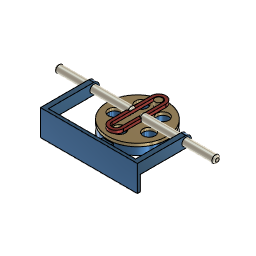
Scotch Yoke (Autodesk Fusion 360 design; units mm, degrees)
Autodesk Fusion 360 part; units mm, degrees
sketch "Sketch1" plane through (0, 0, 0) normal (0, 0, 1) x (1, 0, 0)
  circle A0 centre (0, 0) radius 49
  circle A1 centre (0, 35) radius 6
  line L0 (7, -35) -> (7, 35)
  arc A2 (7, 35) -> (-7, 35) centre (0, 35) ccw
  line L1 (-7, 35) -> (-7, -35)
  arc A3 (-7, -35) -> (7, -35) centre (0, -35) ccw
  line L2 (0, -35) -> (0, 35) construction
  line L3 (12, -35) -> (12, 35)
  arc A4 (12, 35) -> (-12, 35) centre (0, 35) ccw
  line L4 (-12, 35) -> (-12, -35)
  arc A5 (-12, -35) -> (12, -35) centre (0, -35) ccw
  dimension "d1" = 98
  dimension "d2" = 12
  dimension "d3" = 35
  dimension "d4" = 14
  dimension "d5" = 5
  constraint coincident A0.centre origin
  constraint vertical A0.centre A1.centre
  constraint tangent L0 A2
  constraint tangent A2 L1
  constraint parallel L0 L1
  constraint tangent L1 A3
  constraint tangent L0 A3
  constraint coincident A1.centre A2.centre
  constraint vertical L2
  constraint midpoint L2 A0.centre
  measures "d1" diameter of A0
  measures "d2" diameter of A1
  measures "d3" distance of A0.centre A1.centre
  measures "d4" diameter of A2
extrude "Extrude1" add sketch "Sketch1" against normal blind 5 contours A0 | A1 | L0 A2 L1 A3 | L3 A4 L4 A5 makes body 1
extrude "Extrude2" add sketch "Sketch1" along normal blind 10 contours A1 bodies 1
extrude "Extrude3" add sketch "Sketch1" along normal blind 5 separate body contours L3 A4 L4 A5 makes body 2
move_body "Align1" bodies 2 to x (1, 0, 0) y (0, 1, 0) z (0, 0, 1) at (0, 0, 5)
sketch "Sketch2" plane through (12, 0, 0) normal (1, 0, 0) x (0, 1, 0)
  line L0 (-35, 5) -> (35, 5)
  line L1 (35, 5) -> (35, 10)
  line L2 (35, 10) -> (-35, 10)
  line L3 (-35, 10) -> (-35, 5)
  line L4 (0, 5) -> (0, 7.5)
  circle A0 centre (0, 7.5) radius 6
  dimension "d12" = 2.5
  dimension "d13" = 12
  constraint midpoint L0 L4.start
  constraint perpendicular L2 L4
  constraint coincident L4.end A0.centre
  measures "d12" distance of L4.start L4.end
  measures "d13" diameter of A0
extrude "Extrude4" add sketch "Sketch2" along normal blind 60 separate body contours L0 L2 A0 | L0 A0 | L2 A0 makes body 3
extrude "Extrude5" add sketch "Sketch2" against normal blind 5 contours L0 A0 | L2 A0 bodies 3
fillet "Fillet1" radius 3 2 edges at (7, 0, 13.5) (7, 0, 1.5) on bodies 3
sketch "Sketch3" plane through (72, 0, 0) normal (1, 0, 0) x (0, 1, 0)
  circle A0 centre (0, 7.5) radius 6
  circle A1 centre (0, 7.5) radius 6.5
  line L0 (-9, 7.5) -> (-9, -20)
  arc A2 (-9, -20) -> (9, -20) centre (0, -20) ccw
  line L1 (9, -20) -> (9, 7.5)
  arc A3 (9, 7.5) -> (-9, 7.5) centre (0, 7.5) ccw
  line L2 (0, 7.5) -> (0, -20) construction
  line L3 (25, -17.5884) -> (-25, -17.5884)
  line L4 (-25, -17.5884) -> (-25, -8.5884)
  line L5 (-25, -8.5884) -> (25, -8.5884)
  line L6 (25, -8.5884) -> (25, -17.5884)
  line L7 (25, -17.5884) -> (-25, -8.5884) construction
  line L8 (-25, -17.5884) -> (25, -8.5884) construction
  point P0 (0, -13.0884)
  dimension "d20" = 13
  dimension "d21" = 18
  dimension "d22" = 50
  dimension "d23" = 9
  constraint concentric A0 A1
  constraint tangent L0 A2
  constraint tangent A2 L1
  constraint parallel L0 L1
  constraint tangent L1 A3
  constraint tangent L0 A3
  constraint vertical L2
  constraint coincident A0.centre A1.centre
  constraint horizontal L3
  constraint perpendicular L3 L4
  constraint parallel L3 L5
  constraint parallel L4 L6
  constraint coincident L7 P0
  constraint coincident L8 P0
  constraint coincident L2 P0
  measures "d20" diameter of A1
  measures "d21" diameter of A2
  measures "d22" distance of L4.end L5.end
  measures "d23" distance of L3.end L4.end
extrude "Extrude6" add sketch "Sketch3" along normal blind 8 separate body contours L0 L1 A3 L5 | L0 L1 L3 L5 | L0 L3 L4 L5 | L1 L3 L5 L6 makes body 4
extrude "Extrude7" add 1 faces at (72, 1.1757, 4.8674) along direction (1, 0, 0) blind 60 on bodies 3 bodies 3
fillet "Fillet2" radius 3 1 edges at (132, -5.594, 5.3303) on bodies 3
mirror "Mirror1" about plane through (0, 0, 0) normal (1, 0, 0) of bodies 3 4 makes body 5 at (-51.3333, 0, 1.5) makes body 6 at (-72, 0.1619, -5.3862)
sketch "Sketch4" plane through (0, 0, 0) normal (0, 0, 1) x (-1, 0, 0)
  circle A0 centre (0, -35) radius 6
  circle A1 centre (0, 0) radius 49
  circle A2 centre (0, 30) radius 10
  dimension "d32" = 20
  measures "d32" diameter of A2
extrude "Extrude8" cut sketch "Sketch4" against normal blind 100 contours A2 bodies 1
pattern_circular "C-Pattern1" count 5 over 360 about axis through (0, 0, 1.75) along (0, 0, 1) of "Extrude8"
extrude "Extrude9" add 1 faces at (-4.2795, 1.1286, -5) along direction (0, 0, -1) blind 12.588 separate body on bodies 1 makes body 7
copy_body "Body->Comp1" bodies 7 removing the originals makes body 8 in component "plate-base"
copy_body "CutPasteBodies1" bodies 4 removing the originals makes body 9 in component "plate-base"
copy_body "CutPasteBodies2" bodies 6 removing the originals makes body 10 in component "plate-base"
copy_body "Body->Comp2" bodies 1 removing the originals makes body 11 in component "plate"
copy_body "Body->Comp3" bodies 2 removing the originals makes body 12 in component "loop"
copy_body "CutPasteBodies1'" bodies 3 5 removing the originals makes body 13 makes body 14 in component "loop"
move_body "Move1" bodies 10 9 to x (1, 0, 0) y (0, 0, -1) z (0, 1, 0) at (0, -10.4116, 7.4116) in component "plate-base"
move_body "Move2" bodies 9 10 to x (1, 0, 0) y (0, 1, 0) z (0, 0, 1) at (0, 5, 0) in component "plate-base"
move_body "Align1'" bodies 10 to x (1, 0, 0) y (0, 1, 0) z (0, 0, 1) at (0, -2.0884, 0.0884) in component "plate-base"
move_body "Align2" bodies 9 to x (1, 0, 0) y (0, 1, 0) z (0, 0, 1) at (0, -2.0884, 0.0884) in component "plate-base"
move_face "OffsetFaces1" offset -16 1 faces at (-74.6667, -19.0884, -17.5) on bodies 10 in component "plate-base"
move_face "OffsetFaces3" offset -16 1 faces at (-74.6667, -22.0884, 32.5) on bodies 10 in component "plate-base"
move_face "OffsetFaces4" offset -16 1 faces at (74.6667, -22.0884, 32.5) on bodies 9 in component "plate-base"
move_face "OffsetFaces5" offset -16 1 faces at (74.6667, -19.0884, -17.5) on bodies 9 in component "plate-base"
extrude "Extrude1'" add 2 faces at (74.6667, -25.0884, 4.5) (-77.3333, -25.0884, 4.5) along direction (0, -1, 0) blind 50 on bodies 9 10 bodies 9 10 in component "plate-base"
sketch "Sketch8" plane through (0, -75.0884, 0) normal (0, -1, 0) x (1, 0, 0)
  line L0 (-74, -1.5) -> (-74, 16.5)
  line L1 (-74, 16.5) -> (-82, 16.5)
  line L2 (-82, 16.5) -> (-82, -1.5)
  line L3 (-82, -1.5) -> (-74, -1.5)
  line L4 (-82, 16.5) -> (77.6925, 16.5)
  line L5 (77.6925, 16.5) -> (77.6925, -1.4738)
  line L6 (77.6925, -1.4738) -> (-82, -1.4738)
  line L7 (-82, -1.4738) -> (-82, 16.5)
  constraint horizontal L4
  constraint vertical L5
  constraint horizontal L6
  constraint vertical L7
  constraint coincident L1.end L2.start
extrude "Extrude2'" add sketch "Sketch8" along normal blind 5 contours L0 L1 L2 L4 L6 L7 | L0 L4 L5 L6 sketch seen with x (1, 0, 0) y (0, 1, 0) z (0, 0, 1) at (2, 0, 0) bodies 9 10 in component "plate-base"
extrude "Extrude3'" add 1 faces at (79.6925, -76.7551, 10.5087) along direction (1, 0, 0) blind 0.308 on bodies 9 bodies 9 in component "plate-base"
extrude "Extrude4'" cut 1 faces at (80.0005, -76.7551, 10.5087) along direction (-1, 0, 0) blind 0.0005 on bodies 9 bodies 9 in component "plate-base"
extrude "Extrude5'" add 1 faces at (24, -78.4218, -1.4738) along direction (0, 0, -1) blind 25 on bodies 9 bodies 9 in component "plate-base"
sketch "Sketch10" plane through (0, 0, -26.4738) normal (0, 0, -1) x (1, 0, 0)
  line L0 (78, 75.0884) -> (78, 80.0884)
  line L1 (78, 80.0884) -> (-82, 80.0884)
  line L2 (-82, 80.0884) -> (-82, 75.0884)
  line L3 (-82, 75.0884) -> (78, 75.0884)
  line L4 (6.4782, 0) -> (-10.4782, 0)
  line L5 (-10.4782, 0) -> (-10.4782, 80.0884)
  line L6 (-10.4782, 160.1769) -> (6.4782, 160.1769)
  line L7 (6.4782, 80.0884) -> (6.4782, 0)
  line L8 (-10.4782, 80.0884) -> (6.4782, 80.0884)
  constraint horizontal L4
  constraint perpendicular L4 L5
  constraint parallel L4 L6
  constraint parallel L5 L7
extrude "Extrude6'" add sketch "Sketch10" against normal blind 20 contours L3 L4 L5 L7 | L1 L3 L5 L7 L8 sketch seen with x (1, 0, 0) y (0, 1, 0) z (0, 0, 1) at (2, 0, 0) bodies 8 9 in component "plate-base"
component "plate-base" placed x (1, 0, 0) y (0, 1, 0) z (0, 0, 1) at (-2, 0, 0)
component "plate" placed x (1, 0, 0) y (0, 1, 0) z (0, 0, 1) at (-2, 0, 0)
component "loop" placed x (1, 0, 0) y (0, 1, 0) z (0, 0, 1) at (-2, 0, 0)
equation "d65 = -4.864E-04 mm"
named bodies: "plate", "loop", "pivot 1", "stand 1", "pivot 2", "stand 2", "plate-base"
